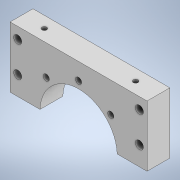
# Autodesk Inventor part: ShooterSeperableClampB
Saved by Autodesk Inventor 2020 (Build 240168000, 168)
## iProperties
Created: 2020-01-29
Part Number: ShooterSeperableClampB
Material: Generic
Document SubType Name: Modeling
Designer: srini
Density: 1 g/cm^3
Appearance: Default
Author: srini
Autodesk Inventor part; units mm, degrees
ref_plane "YZ Plane" through (0, 0, 0) normal (1, 0, 0) x (0, 1, 0)
ref_plane "XZ Plane" through (0, 0, 0) normal (0, 1, 0) x (-1, 0, 0)
ref_plane "XY Plane" through (0, 0, 0) normal (0, 0, 1) x (1, 0, 0)
sketch "Sketch1" plane through (0, 0, 0) normal (0, 0, 1) x (1, 0, 0)
  line L0 (57.15, -25.4) -> (-57.15, -25.4)
  line L1 (-57.15, -25.4) -> (-57.15, 25.4)
  line L2 (-57.15, 25.4) -> (57.15, 25.4)
  line L3 (57.15, 25.4) -> (57.15, -25.4)
  line L4 (57.15, -25.4) -> (-57.15, 25.4) construction
  line L5 (-57.15, -25.4) -> (57.15, 25.4) construction
  point P0 (0, 0)
  dimension "d0" = 50.8
  dimension "d1" = 114.3
  constraints: 12 end point, 2 midpoint, 2 parallel, 1 horizontal, 1 perpendicular
  measures "d0" distance of L0.end L1.end
  measures "d1" distance of L1.end L2.end
extrude "Extrusion1" add sketch "Sketch1" along normal blind 19.05
sketch "Sketch2" plane through (0, 0, 19.05) normal (0, 0, 1) x (1, 0, 0)
  circle A0 centre (-50.8, 15.875) radius 3.3734
  line L0 (57.15, 25.4) -> (-57.15, 25.4) projected
  line L1 (-57.15, 25.4) -> (-57.15, -25.4) projected
  circle A1 centre (50.8, 15.875) radius 3.3734
  circle A2 centre (-50.8, -9.525) radius 3.3734
  circle A3 centre (50.8, -9.525) radius 3.3734
  circle A4 centre (0, -26.67) radius 32.258
  line L2 (-57.15, -25.4) -> (57.15, -25.4) projected
  point P0 (0, 0)
  dimension "d4" = 50.8
  dimension "d5" = 9.525
  dimension "d6" = 6.7469
  dimension "d9" = 101.6
  dimension "d12" = 25.4
  dimension "d15" = 1.27
  dimension "d16" = 64.516
  constraints: 5 centre point, 1 horizontal, 1 vertical, 1 vertical alignment, 6 other
  measures "d4" horizontal distance of A0.centre point (0, 0)
  measures "d5" distance from line of A0.centre L0
  measures "d6" diameter of A0
  measures "d9" distance of A0.centre A1.centre
  measures "d12" distance of A0.centre A2.centre
  measures "d15" distance from line of A4.centre L2
  measures "d16" diameter of A4
extrude "Extrusion2" cut sketch "Sketch2" against normal through all
sketch "Sketch3" plane through (-57.15, 25.4, 0) normal (0, 1, 0) x (1, 0, 0)
  circle A0 centre (19.05, -9.525) radius 2.0193
  line L0 (114.3, 0) -> (0, 0) projected
  circle A1 centre (95.25, -9.525) radius 2.0193
  point P0 (57.15, 0)
  dimension "d19" = 4.0386
  dimension "d20" = 9.525
  dimension "d21" = 38.1
  dimension "d24" = 76.2
  constraints: 2 centre point, 1 horizontal, 2 other
  measures "d19" diameter of A0
  measures "d20" distance from line of A0.centre L0
  measures "d21" horizontal distance of A0.centre point (57.15, 0)
  measures "d24" distance of A0.centre A1.centre
extrude "Extrusion3" cut sketch "Sketch3" against normal through all
sketch "Sketch4" plane through (0, 0, 19.05) normal (0, 0, 1) x (1, 0, 0)
  circle A0 centre (-26.9408, 0.2708) radius 2.5797
  arc A1 (32.233, -25.4) -> (-32.233, -25.4) centre (0, -26.67) ccw projected
  circle A2 centre (0, 11.43) radius 2.5797
  circle A3 centre (26.9408, 0.2708) radius 2.5797
  point P0 (0, 0)
  dimension "d31" = 5.1594
  dimension "d32" = 38.1
  dimension "d33" = 45
  dimension "d36" = 90
  constraints: 3 centre point, 5 other
  measures "d31" diameter of A0
  measures "d32" distance of A0.centre A1.centre
extrude "Extrusion4" cut sketch "Sketch4" against normal through all
body "Solid1"
